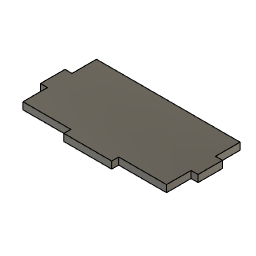
Assemble_Habits v10 (Autodesk Fusion 360 archive; units mm, degrees)
design "tray_front2_43x25_trans_2mm"
Autodesk Fusion 360 part; units mm, degrees
note: some values were not read from the file. Set by a fixed rule: which face or edge a step refers to.
(part 1 of 2)
sketch "Sketch1" plane through (0, 0, 0) normal (0, 0, 1) x (1, 0, 0)
  line L0 (0, 0) -> (41, 0)
  line L1 (41, 0) -> (41, -21)
  line L2 (41, -21) -> (0, -21)
  line L3 (0, -21) -> (0, 0)
  line L4 (0, -21) -> (0, -14)
  line L5 (0, -14) -> (-2, -14)
  line L6 (-2, -14) -> (-2, -7)
  line L7 (-2, -7) -> (0, -7)
  line L8 (0, -7) -> (0, -14)
  line L9 (41, -21) -> (41, -14)
  line L10 (41, -14) -> (43, -14)
  line L11 (43, -14) -> (43, -7)
  line L12 (43, -7) -> (41, -7)
  line L13 (41, -7) -> (41, -14)
  line L14 (0, -21) -> (13.67, -21)
  line L15 (13.67, -21) -> (27.34, -21)
  line L16 (27.34, -21) -> (27.34, -23)
  line L17 (27.34, -23) -> (13.67, -23)
  line L18 (13.67, -23) -> (13.67, -21)
  dimension "d1" = 41
  dimension "d2" = 21
  dimension "d5" = 7
  dimension "d6" = 2
  dimension "d7" = 7
  dimension "d8" = 7
  dimension "d9" = 2
  dimension "d10" = 7
  dimension "d11" = 13.67
  dimension "d12" = 13.67
  dimension "d13" = 2
  constraint horizontal L0
  constraint vertical L1
  constraint horizontal L2
  constraint vertical L3
  constraint coincident L0.start L3.end
  constraint perpendicular L2 L4
  constraint horizontal L5
  constraint vertical L6
  constraint horizontal L7
  constraint vertical L8
  constraint perpendicular L2 L9
  constraint horizontal L10
  constraint vertical L11
  constraint horizontal L12
  constraint vertical L13
  constraint perpendicular L3 L14
  constraint horizontal L15
  constraint vertical L16
  constraint horizontal L17
  constraint vertical L18
  measures "d1" distance of L0.start L0.end
  measures "d2" distance of L0.start L2.end
  measures "d5" distance of L2.end L4.end
  measures "d6" distance of L4.end L5.end
  measures "d7" distance of L4.end L7.end
  measures "d8" distance of L1.end L9.end
  measures "d9" distance of L9.end L10.end
  measures "d10" distance of L9.end L12.end
  measures "d11" distance of L2.end L14.end
  measures "d12" distance of L14.end L15.end
  measures "d13" distance of L14.end L17.end
extrude "Extrude1" add sketch "Sketch1" along normal blind 2

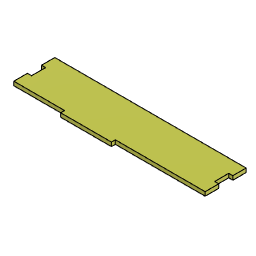
design "tray_side2_98x23_trans_2mm"
Autodesk Fusion 360 part; units mm, degrees
sketch "Sketch1" plane through (0, 0, 0) normal (0, 0, 1) x (1, 0, 0)
  line L0 (0, 0) -> (98, 0)
  line L1 (98, 0) -> (98, -21)
  line L2 (98, -21) -> (0, -21)
  line L3 (0, -21) -> (0, 0)
  line L4 (0, -21) -> (0, -14)
  line L5 (0, -14) -> (2.1, -14)
  line L6 (2.1, -14) -> (2.1, -6.8)
  line L7 (2.1, -6.8) -> (0, -6.8)
  line L8 (0, -6.8) -> (0, -14)
  line L9 (98, -21) -> (98, -14)
  line L10 (98, -14) -> (95.9, -14)
  line L11 (95.9, -14) -> (95.9, -6.8)
  line L12 (95.9, -6.8) -> (98, -6.8)
  line L13 (98, -6.8) -> (98, -14)
  line L14 (0, -21) -> (26, -21)
  line L15 (26, -21) -> (52, -21)
  line L16 (52, -21) -> (52, -23)
  line L17 (52, -23) -> (26, -23)
  line L18 (26, -23) -> (26, -21)
  dimension "d1" = 98
  dimension "d2" = 21
  dimension "d5" = 7
  dimension "d6" = 2.1
  dimension "d7" = 7.2
  dimension "d8" = 7
  dimension "d9" = 2.1
  dimension "d10" = 7.2
  dimension "d11" = 26
  dimension "d12" = 26
  dimension "d13" = 2
  constraint horizontal L0
  constraint vertical L1
  constraint horizontal L2
  constraint vertical L3
  constraint coincident L0.start L3.end
  constraint perpendicular L2 L4
  constraint horizontal L5
  constraint vertical L6
  constraint horizontal L7
  constraint vertical L8
  constraint perpendicular L2 L9
  constraint horizontal L10
  constraint vertical L11
  constraint horizontal L12
  constraint vertical L13
  constraint perpendicular L3 L14
  constraint horizontal L15
  constraint vertical L16
  constraint horizontal L17
  constraint vertical L18
  measures "d1" distance of L0.start L0.end
  measures "d2" distance of L0.start L2.end
  measures "d5" distance of L2.end L4.end
  measures "d6" distance of L4.end L5.end
  measures "d7" distance of L4.end L7.end
  measures "d8" distance of L1.end L9.end
  measures "d9" distance of L9.end L10.end
  measures "d10" distance of L9.end L12.end
  measures "d11" distance of L2.end L14.end
  measures "d12" distance of L14.end L15.end
  measures "d13" distance of L14.end L17.end
extrude "Extrude1" add sketch "Sketch1" along normal blind 2 contours L0 L1 L2 L3 L4 L5 L6 L7 L9 L10 L11 L12 L14 L15 | L2 L15 L16 L17 L18

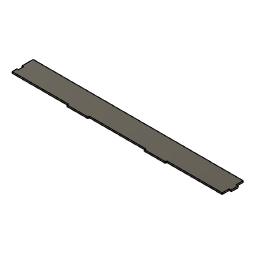
design "tray_side_302x32_trans_2mm"
Autodesk Fusion 360 part; units mm, degrees
sketch "Sketch1" plane through (0, 0, 0) normal (0, 0, 1) x (1, 0, 0)
  line L0 (0, 0) -> (299, 0)
  line L1 (299, 0) -> (299, -30)
  line L2 (299, -30) -> (0, -30)
  line L3 (0, -30) -> (0, 0)
  line L4 (0, -30) -> (0, -23)
  line L5 (0, -23) -> (2.1, -23)
  line L6 (2.1, -23) -> (2.1, -15.8)
  line L7 (2.1, -15.8) -> (0, -15.8)
  line L8 (0, -15.8) -> (0, -23)
  line L9 (299, -30) -> (299, -20)
  line L10 (299, -20) -> (302, -20)
  line L11 (302, -20) -> (302, -10)
  line L12 (302, -10) -> (299, -10)
  line L13 (299, -10) -> (299, -20)
  line L14 (0, -30) -> (80, -30)
  line L15 (80, -30) -> (110, -30)
  line L16 (110, -30) -> (110, -32)
  line L17 (110, -32) -> (80, -32)
  line L18 (80, -32) -> (80, -30)
  line L19 (110, -30) -> (190.2, -30)
  line L20 (190.2, -30) -> (220.2, -30)
  line L21 (220.2, -30) -> (220.2, -32)
  line L22 (220.2, -32) -> (190.2, -32)
  line L23 (190.2, -32) -> (190.2, -30)
  dimension "d1" = 299
  dimension "d2" = 30
  dimension "d5" = 7
  dimension "d6" = 2.1
  dimension "d7" = 7.2
  dimension "d8" = 10
  dimension "d9" = 3
  dimension "d10" = 10
  dimension "d11" = 80
  dimension "d12" = 30
  dimension "d13" = 2
  dimension "d14" = 80.2
  dimension "d15" = 30
  dimension "d16" = 2
  constraint horizontal L0
  constraint vertical L1
  constraint horizontal L2
  constraint vertical L3
  constraint coincident L0.start L3.end
  constraint perpendicular L2 L4
  constraint horizontal L5
  constraint vertical L6
  constraint horizontal L7
  constraint vertical L8
  constraint perpendicular L2 L9
  constraint horizontal L10
  constraint vertical L11
  constraint horizontal L12
  constraint vertical L13
  constraint perpendicular L4 L14
  constraint horizontal L15
  constraint vertical L16
  constraint horizontal L17
  constraint vertical L18
  constraint perpendicular L16 L19
  constraint horizontal L20
  constraint vertical L21
  constraint horizontal L22
  constraint vertical L23
  measures "d1" distance of L0.start L0.end
  measures "d2" distance of L0.start L2.end
  measures "d5" distance of L2.end L4.end
  measures "d6" distance of L4.end L5.end
  measures "d7" distance of L4.end L7.end
  measures "d8" distance of L1.end L9.end
  measures "d9" distance of L9.end L10.end
  measures "d10" distance of L9.end L12.end
  measures "d11" distance of L2.end L14.end
  measures "d12" distance of L14.end L15.end
  measures "d13" distance of L14.end L17.end
  measures "d14" distance of L15.end L19.end
  measures "d15" distance of L19.end L20.end
  measures "d16" distance of L19.end L22.end
extrude "Extrude1" add sketch "Sketch1" along normal blind 2 contours L0 L1 L2 L3 L4 L5 L6 L7 L9 L13 L14 L15 L19 L20 | L1 L10 L11 L12 L13 | L2 L15 L16 L17 L18 | L2 L20 L21 L22 L23

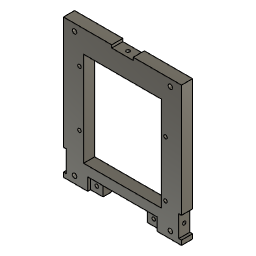
design "Front_holder"
Autodesk Fusion 360 part; units mm, degrees
sketch "Sketch1" plane through (0, 0, 0) normal (0, 1, 0) x (1, 0, 0)
  line L0 (0, 0) -> (85, 0)
  line L1 (85, 0) -> (85, -100)
  line L2 (85, -100) -> (0, -100)
  line L3 (0, -100) -> (0, 0)
  line L4 (85, 0) -> (85, -3.25)
  line L5 (85, -3.25) -> (83, -3.25)
  line L6 (83, -3.25) -> (83, -18.75)
  line L7 (83, -18.75) -> (85, -18.75)
  line L8 (85, -18.75) -> (85, -3.25)
  line L9 (0, 0) -> (0, -3.25)
  line L10 (0, -3.25) -> (2, -3.25)
  line L11 (2, -3.25) -> (2, -18.75)
  line L12 (2, -18.75) -> (0, -18.75)
  line L13 (0, -18.75) -> (0, -3.25)
  line L14 (0, -100) -> (34.75, -100)
  line L15 (34.75, -100) -> (50.25, -100)
  line L16 (50.25, -100) -> (50.25, -98)
  line L17 (50.25, -98) -> (34.75, -98)
  line L18 (34.75, -98) -> (34.75, -100)
  line L19 (0, -100) -> (8.5, -100)
  line L20 (8.5, -100) -> (8.5, -90)
  line L21 (8.5, -90) -> (0, -90)
  line L22 (0, -90) -> (0, -100)
  line L23 (8.5, -90) -> (76.5, -90)
  line L24 (76.5, -90) -> (76.5, -10)
  line L25 (76.5, -10) -> (8.5, -10)
  line L26 (8.5, -10) -> (8.5, -90)
  circle A0 centre (8, -95) radius 1.6
  circle A1 centre (77, -95) radius 1.6
  circle A2 centre (8, -5) radius 1.6
  circle A3 centre (77, -5) radius 1.6
  circle A4 centre (11.5, -35) radius 1.25
  circle A5 centre (11.5, -75) radius 1.25
  circle A6 centre (73.5, -22) radius 1.25
  line L27 (8.5, -90) -> (14.5, -90)
  line L28 (14.5, -90) -> (14.5, -84)
  line L29 (14.5, -84) -> (8.5, -84)
  line L30 (8.5, -84) -> (8.5, -90)
  line L31 (14.5, -84) -> (70.5, -84)
  line L32 (70.5, -84) -> (70.5, -16)
  line L33 (70.5, -16) -> (14.5, -16)
  line L34 (14.5, -16) -> (14.5, -84)
  circle A7 centre (73.5, -62) radius 1.25
  line L35 (42.5, 0) -> (67.5, 0)
  line L36 (67.5, 0) -> (17.5, 0)
  line L37 (17.5, 0) -> (17.5, -9)
  line L38 (17.5, -9) -> (67.5, -9)
  line L39 (67.5, -9) -> (67.5, 0)
  line L40 (17.5, 0) -> (26.5, 0)
  line L41 (67.5, 0) -> (58.5, 0)
  line L42 (26.5, 0) -> (26.5, -9)
  line L43 (58.5, 0) -> (58.5, -9)
  circle A8 centre (22, -4.5) radius 1.25
  circle A9 centre (63, -4.5) radius 1.25
  dimension "d1" = 85
  dimension "d2" = 100
  dimension "d25" = 3.25
  dimension "d26" = 2
  dimension "d27" = 15.5
  dimension "d28" = 3.25
  dimension "d29" = 2
  dimension "d30" = 15.5
  dimension "d31" = 34.75
  dimension "d32" = 15.5
  dimension "d33" = 2
  dimension "d45" = 8.5
  dimension "d46" = 10
  dimension "d47" = 68
  dimension "d48" = 80
  dimension "d49" = 3.2
  dimension "d50" = 8
  dimension "d51" = 3.2
  dimension "d52" = 8
  dimension "d53" = 3.2
  dimension "d54" = 5
  dimension "d55" = 3.2
  dimension "d56" = 8
  dimension "d57" = 2.5
  dimension "d58" = 25
  dimension "d59" = 3
  dimension "d60" = 2.5
  dimension "d61" = 65
  dimension "d62" = 2.5
  dimension "d63" = 65
  dimension "d64" = 12
  dimension "d161" = 6
  dimension "d162" = 6
  dimension "d163" = 56
  dimension "d164" = 68
  dimension "d167" = 8
  dimension "d168" = 5
  dimension "d213" = 2.5
  dimension "d214" = 40
  dimension "d215" = 25
  dimension "d216" = 50
  dimension "d217" = 9
  dimension "d218" = 9
  dimension "d219" = 9
  dimension "d223" = 2.5
  dimension "d224" = 2.5
  dimension "d225" = 4.5
  dimension "d226" = 4.5
  constraint horizontal L0
  constraint vertical L1
  constraint horizontal L2
  constraint vertical L3
  constraint coincident L0.start L3.end
  constraint perpendicular L0 L4
  constraint horizontal L5
  constraint vertical L6
  constraint horizontal L7
  constraint vertical L8
  constraint perpendicular L0 L9
  constraint horizontal L10
  constraint vertical L11
  constraint horizontal L12
  constraint vertical L13
  constraint perpendicular L3 L14
  constraint horizontal L15
  constraint vertical L16
  constraint horizontal L17
  constraint vertical L18
  constraint horizontal L19
  constraint vertical L20
  constraint horizontal L21
  constraint vertical L22
  constraint horizontal L23
  constraint vertical L24
  constraint horizontal L25
  constraint vertical L26
  constraint horizontal L27
  constraint vertical L28
  constraint horizontal L29
  constraint vertical L30
  constraint horizontal L31
  constraint vertical L32
  constraint horizontal L33
  constraint vertical L34
  constraint midpoint L0 L35.start
  constraint parallel L0 L35
  constraint horizontal L36
  constraint vertical L37
  constraint horizontal L38
  constraint vertical L39
  constraint perpendicular L37 L40
  constraint perpendicular L39 L41
  constraint coincident L38 L42.end
  constraint perpendicular L38 L42
  constraint coincident L38 L43.end
  constraint perpendicular L38 L43
  measures "d1" distance of L0.start L0.end
  measures "d2" distance of L0.start L2.end
  measures "d25" distance of L0.end L4.end
  measures "d26" distance of L4.end L5.end
  measures "d27" distance of L4.end L7.end
  measures "d28" distance of L0.start L9.end
  measures "d29" distance of L9.end L10.end
  measures "d30" distance of L9.end L12.end
  measures "d31" distance of L2.end L14.end
  measures "d32" distance of L14.end L15.end
  measures "d33" distance of L14.end L17.end
  measures "d45" distance of L2.end L19.end
  measures "d46" distance of L2.end L21.end
  measures "d47" distance of L20.end L23.end
  measures "d48" distance of L20.end L25.end
  measures "d49" diameter of A0
  measures "d50" distance of L3 A0.centre
  measures "d51" diameter of A1
  measures "d52" distance of L1 A1.centre
  measures "d53" diameter of A2
  measures "d54" distance of L0 A2.centre
  measures "d55" diameter of A3
  measures "d56" distance of L8 A3.centre
  measures "d57" diameter of A4
  measures "d58" distance of L25 A4.centre
  measures "d59" distance of L26 A4.centre
  measures "d60" diameter of A5
  measures "d61" distance of L25 A5.centre
  measures "d62" diameter of A6
  measures "d63" distance of L26 A6.centre
  measures "d64" distance of L25 A6.centre
  measures "d161" distance of L20.end L27.end
  measures "d162" distance of L20.end L29.end
  measures "d163" distance of L28.end L31.end
  measures "d164" distance of L28.end L33.end
  measures "d167" distance of L13 A2.centre
  measures "d168" distance of L0 A3.centre
  measures "d213" diameter of A7
  measures "d214" distance of A6.centre A7.centre
  measures "d215" distance of L35.start L35.end
  measures "d216" distance of L35.end L36.end
  measures "d217" distance of L35.end L38.end
  measures "d218" distance of L36.end L40.end
  measures "d219" distance of L35.end L41.end
  measures "d223" diameter of A8
  measures "d224" diameter of A9
  measures "d225" distance of L37 A8.centre
  measures "d226" distance of L39 A9.centre
extrude "Extrude1" add sketch "Sketch1" along normal blind 8 contours L23 L26 L27 L28 L29 L30 | L0 L1 L2 L3 L4 L5 L6 L7 L9 L10 L11 L12 L14 L16 L17 L18 L20 L21 A0 L37 L38 L39 | L2 L3 L14 L19 L20 L21 L22 A0 | L23 L24 L25 L26 L28 L29
hole "Hole1" at (42.5, 4, 98) direction (0, 0, -1) diameter 2.5 depth 12 tip angle 180
hole "Hole2" at (83, 4, 11) direction (-1, 0, 0) diameter 2.5 depth 12 tip angle 180
hole "Hole3" at (2, 4, 11) direction (1, 0, 0) diameter 2.5 depth 12 tip angle 180
extrude "Extrude7" add sketch "Sketch1" along normal blind 6 from surface at 2 contours L0 L36 L37 L38 L40 L42 | L0 L35 L36 L38 L39 L41 L43

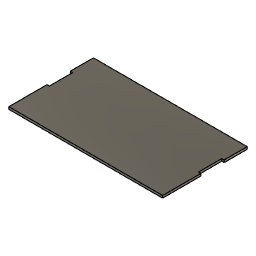
design "cage_back_200x110_trans_3mm"
Autodesk Fusion 360 part; units mm, degrees
sketch "Sketch1" plane through (0, 0, 0) normal (0, 0, 1) x (1, 0, 0)
  line L0 (0, 0) -> (200, 0)
  line L1 (200, 0) -> (200, -110)
  line L2 (200, -110) -> (0, -110)
  line L3 (0, -110) -> (0, 0)
  line L4 (0, 0) -> (0, -30)
  line L5 (0, -30) -> (3.1, -30)
  line L6 (3.1, -30) -> (3.1, -60.2)
  line L7 (3.1, -60.2) -> (0, -60.2)
  line L8 (0, -60.2) -> (0, -30)
  line L9 (200, 0) -> (200, -30)
  line L10 (200, -30) -> (196.9, -30)
  line L11 (196.9, -30) -> (196.9, -60.2)
  line L12 (196.9, -60.2) -> (200, -60.2)
  line L13 (200, -60.2) -> (200, -30)
  dimension "d1" = 200
  dimension "d2" = 110
  dimension "d5" = 30
  dimension "d6" = 3.1
  dimension "d7" = 30.2
  dimension "d8" = 30
  dimension "d9" = 3.1
  dimension "d10" = 30.2
  constraint horizontal L0
  constraint vertical L1
  constraint horizontal L2
  constraint vertical L3
  constraint coincident L0.start L3.end
  constraint parallel L3 L4
  constraint horizontal L5
  constraint vertical L6
  constraint horizontal L7
  constraint vertical L8
  constraint perpendicular L0 L9
  constraint horizontal L10
  constraint vertical L11
  constraint horizontal L12
  constraint vertical L13
  measures "d1" distance of L0.start L0.end
  measures "d2" distance of L0.start L2.end
  measures "d5" distance of L0.start L4.end
  measures "d6" distance of L4.end L5.end
  measures "d7" distance of L4.end L7.end
  measures "d8" distance of L0.end L9.end
  measures "d9" distance of L9.end L10.end
  measures "d10" distance of L9.end L12.end
extrude "Extrude1" add sketch "Sketch1" along normal blind 3 contours L0 L1 L2 L3 L4 L5 L6 L7 L9 L10 L11 L12

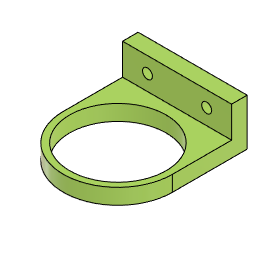
design "Tube_holder"
Autodesk Fusion 360 part; units mm, degrees
sketch "Sketch1" plane through (0, 0, 0) normal (0, 0, 1) x (1, 0, 0)
  circle A0 centre (0, 0) radius 15.5
  circle A1 centre (0, 0) radius 17.5
  line L0 (0, 0) -> (17.5, 0)
  line L1 (0, 0) -> (-17.5, 0)
  line L2 (-17.5, 0) -> (-17.5, 24)
  line L3 (17.5, 0) -> (17.5, 24)
  line L4 (-17.5, 24) -> (17.5, 24)
  line L5 (-17.5, 24) -> (-17.5, 19)
  line L6 (-17.5, 19) -> (17.5, 19)
  dimension "d1" = 31
  dimension "d2" = 35
  dimension "d3" = 24
  dimension "d4" = 24
  dimension "d9" = 5
  constraint coincident A0.centre A1.centre
  constraint concentric A0 A1
  constraint coincident A1 L0.end
  constraint horizontal L0
  constraint coincident A1 L1.end
  constraint parallel L0 L1
  constraint perpendicular L1 L2
  constraint perpendicular L0 L3
  constraint perpendicular L4 L5
  constraint coincident L3 L6.end
  constraint perpendicular L3 L6
  measures "d1" diameter of A0
  measures "d2" diameter of A1
  measures "d3" distance of L1.end L2.end
  measures "d4" distance of L0.end L3.end
  measures "d9" distance of L2.end L5.end
extrude "Extrude1" add sketch "Sketch1" along normal blind 5 contours A0 A1 L0 L1 | A0 A1 L0 L1 | A1 L2 L3 L6 | L2 L3 L4 L5 L6
extrude "Extrude2" add sketch "Sketch1" along normal blind 15 contours L2 L3 L4 L5 L6
sketch "Sketch2" plane through (0, 19, 0) normal (0, -1, 0) x (1, 0, 0)
  line L0 (-17.5, 5) -> (17.5, 5)
  line L1 (17.5, 5) -> (17.5, 15)
  line L2 (17.5, 15) -> (-17.5, 15)
  line L3 (-17.5, 15) -> (-17.5, 5)
  circle A0 centre (-9.5, 10) radius 1.6
  circle A1 centre (9.5, 10) radius 1.6
  dimension "d10" = 3.2
  dimension "d11" = 3.2
  dimension "d12" = 8
  dimension "d13" = 8
  measures "d10" diameter of A0
  measures "d11" diameter of A1
  measures "d12" distance of L3 A0.centre
  measures "d13" distance of L1 A1.centre
extrude "Extrude3" cut sketch "Sketch2" against normal blind 5 contours A0 | A1

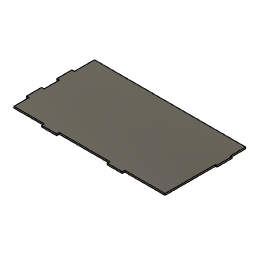
design "cage_side_308x165_blk_3mm"
Autodesk Fusion 360 part; units mm, degrees
sketch "Sketch1" plane through (0, 0, 0) normal (0, 0, 1) x (1, 0, 0)
  line L0 (0, 0) -> (300, 0)
  line L1 (300, 0) -> (300, -160)
  line L2 (300, -160) -> (0, -160)
  line L3 (0, -160) -> (0, 0)
  line L4 (0, -160) -> (60, -160)
  line L5 (60, -160) -> (90, -160)
  line L6 (90, -160) -> (90, -165)
  line L7 (90, -165) -> (60, -165)
  line L8 (60, -165) -> (60, -160)
  line L9 (90, -160) -> (190.2, -160)
  line L10 (190.2, -160) -> (220.2, -160)
  line L11 (220.2, -160) -> (220.2, -165)
  line L12 (220.2, -165) -> (190.2, -165)
  line L13 (190.2, -165) -> (190.2, -160)
  line L14 (0, -160) -> (0, -130)
  line L15 (0, -130) -> (-5, -130)
  line L16 (-5, -130) -> (-5, -100)
  line L17 (-5, -100) -> (0, -100)
  line L18 (0, -100) -> (0, -130)
  line L19 (0, -100) -> (0, -69.8)
  line L20 (0, -69.8) -> (-5, -69.8)
  line L21 (-5, -69.8) -> (-5, -39.8)
  line L22 (-5, -39.8) -> (0, -39.8)
  line L23 (0, -39.8) -> (0, -69.8)
  line L24 (300, 0) -> (300, -30)
  line L25 (300, -30) -> (303, -30)
  line L26 (303, -30) -> (303, -60)
  line L27 (303, -60) -> (300, -60)
  line L28 (300, -60) -> (300, -30)
  dimension "d1" = 300
  dimension "d2" = 160
  dimension "d5" = 60
  dimension "d6" = 30
  dimension "d7" = 5
  dimension "d8" = 100.2
  dimension "d9" = 30
  dimension "d10" = 5
  dimension "d11" = 30
  dimension "d12" = 5
  dimension "d13" = 30
  dimension "d14" = 30.2
  dimension "d15" = 5
  dimension "d16" = 30
  dimension "d17" = 30
  dimension "d18" = 3
  dimension "d19" = 30
  constraint horizontal L0
  constraint vertical L1
  constraint horizontal L2
  constraint vertical L3
  constraint coincident L0.start L3.end
  constraint perpendicular L3 L4
  constraint horizontal L5
  constraint vertical L6
  constraint horizontal L7
  constraint vertical L8
  constraint perpendicular L6 L9
  constraint horizontal L10
  constraint vertical L11
  constraint horizontal L12
  constraint vertical L13
  constraint perpendicular L4 L14
  constraint horizontal L15
  constraint vertical L16
  constraint horizontal L17
  constraint vertical L18
  constraint perpendicular L17 L19
  constraint horizontal L20
  constraint vertical L21
  constraint horizontal L22
  constraint vertical L23
  constraint perpendicular L0 L24
  constraint horizontal L25
  constraint vertical L26
  constraint horizontal L27
  constraint vertical L28
  measures "d1" distance of L0.start L0.end
  measures "d2" distance of L0.start L2.end
  measures "d5" distance of L2.end L4.end
  measures "d6" distance of L4.end L5.end
  measures "d7" distance of L4.end L7.end
  measures "d8" distance of L5.end L9.end
  measures "d9" distance of L9.end L10.end
  measures "d10" distance of L9.end L12.end
  measures "d11" distance of L2.end L14.end
  measures "d12" distance of L14.end L15.end
  measures "d13" distance of L14.end L17.end
  measures "d14" distance of L17.end L19.end
  measures "d15" distance of L19.end L20.end
  measures "d16" distance of L19.end L22.end
  measures "d17" distance of L0.end L24.end
  measures "d18" distance of L24.end L25.end
  measures "d19" distance of L24.end L27.end
extrude "Extrude1" add sketch "Sketch1" along normal blind 3

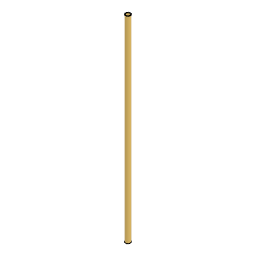
design "Lickport"
Autodesk Fusion 360 part; units mm, degrees
sketch "Sketch1" plane through (0, 0, 0) normal (0, 0, 1) x (1, 0, 0)
  circle A0 centre (0, 0) radius 0.75
  circle A1 centre (0, 0) radius 0.6
  dimension "d1" = 1.5
  dimension "d4" = 1.2
  constraint coincident A0.centre A1.centre
  constraint concentric A0 A1
  measures "d1" diameter of A0
  measures "d4" diameter of A1
extrude "Extrude2" add sketch "Sketch1" along normal blind 60

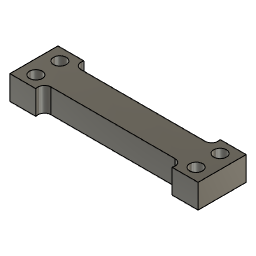
design "weight_Load cell"
Autodesk Fusion 360 part; units mm, degrees
sketch "Sketch1" plane through (0, 0, 0) normal (0, 0, 1) x (1, 0, 0)
  line L0 (0, 0) -> (47, 0)
  line L1 (47, 0) -> (47, -12)
  line L2 (47, -12) -> (0, -12)
  line L3 (0, -12) -> (0, 0)
  circle A0 centre (3.5, -3) radius 1.6
  circle A1 centre (3.5, -9) radius 1.6
  circle A2 centre (43.5, -3) radius 1.6
  circle A3 centre (43.5, -9) radius 1.6
  line L4 (23.5, 0) -> (6.5, 0)
  line L5 (23.5, -2.25) -> (8, -2.25)
  arc A4 (6.5, 0) -> (8, -2.25) centre (8, -0.625) ccw
  line L6 (23.5, -2.25) -> (39, -2.25)
  line L7 (23.5, 0) -> (40.5, 0)
  arc A5 (39, -2.25) -> (40.5, 0) centre (39, -0.625) ccw
  line L8 (23.5, -9.75) -> (8, -9.75)
  line L9 (23.5, -9.75) -> (39, -9.75)
  line L10 (23.5, -12) -> (40.5, -12)
  line L11 (23.5, -12) -> (6.5, -12)
  arc A6 (8, -9.75) -> (6.5, -12) centre (8, -11.375) ccw
  arc A7 (40.5, -12) -> (39, -9.75) centre (39, -11.375) ccw
  dimension "d2" = 47
  dimension "d3" = 12
  dimension "d4" = 40
  dimension "d5" = 6
  dimension "d6" = 3.2
  dimension "d7" = 3.2
  dimension "d8" = 3.2
  dimension "d9" = 3.2
  dimension "d12" = 17
  dimension "d13" = 15.5
  dimension "d14" = 15.5
  dimension "d15" = 17
  dimension "d17" = 15.5
  dimension "d18" = 15.5
  dimension "d19" = 17
  dimension "d20" = 17
  constraint horizontal L0
  constraint vertical L1
  constraint horizontal L2
  constraint vertical L3
  constraint coincident L0.start L3.end
  constraint midpoint L0 L4.start
  constraint parallel L0 L4
  constraint tangent L5 A4
  constraint parallel L0 L7
  constraint tangent L6 A5
  constraint midpoint L2 L10.start
  constraint parallel L2 L10
  constraint parallel L2 L11
  constraint tangent L8 A6
  constraint tangent L9 A7
  measures "d2" distance of L0.start L0.end
  measures "d3" distance of L0.start L2.end
  measures "d4" distance of A0.centre A2.centre
  measures "d5" distance of A0.centre A1.centre
  measures "d6" diameter of A0
  measures "d7" diameter of A1
  measures "d8" diameter of A2
  measures "d9" diameter of A3
  measures "d12" distance of L4.start L4.end
  measures "d13" distance of L5.start L5.end
  measures "d14" distance of L5.start L6.end
  measures "d15" distance of L4.start L7.end
  measures "d17" distance of L8.start L8.end
  measures "d18" distance of L8.start L9.end
  measures "d19" distance of L10.start L10.end
  measures "d20" distance of L10.start L11.end
extrude "Extrude1" add sketch "Sketch1" along normal blind 6 contours L0 L1 L2 L3 L5 A4 L6 A5 L8 L9 A6 A7
equation "d13 = 17 mm - 1.5 mm"

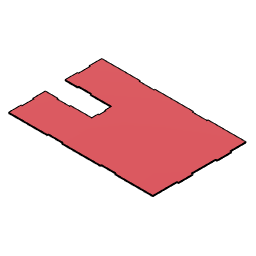
design "tray_bottom_302x193_trans_2mm"
Autodesk Fusion 360 part; units mm, degrees
sketch "Sketch1" plane through (0, 0, 0) normal (0, 0, 1) x (1, 0, 0)
  line L0 (0, 0) -> (299, 0)
  line L1 (299, 0) -> (299, -193)
  line L2 (299, -193) -> (0, -193)
  line L3 (0, -193) -> (0, 0)
  line L4 (0, -193) -> (80, -193)
  line L5 (80, -193) -> (110.2, -193)
  line L6 (110.2, -193) -> (110.2, -190.9)
  line L7 (110.2, -190.9) -> (80, -190.9)
  line L8 (80, -190.9) -> (80, -193)
  line L9 (110.2, -193) -> (190.2, -193)
  line L10 (190.2, -193) -> (220.4, -193)
  line L11 (220.4, -193) -> (220.4, -190.9)
  line L12 (220.4, -190.9) -> (190.2, -190.9)
  line L13 (190.2, -190.9) -> (190.2, -193)
  line L14 (0, 0) -> (80, 0)
  line L15 (80, 0) -> (110.2, 0)
  line L16 (110.2, 0) -> (110.2, -2.1)
  line L17 (110.2, -2.1) -> (80, -2.1)
  line L18 (80, -2.1) -> (80, 0)
  line L19 (110.2, 0) -> (190.2, 0)
  line L20 (190.2, 0) -> (220.4, 0)
  line L21 (220.4, 0) -> (220.4, -2.1)
  line L22 (220.4, -2.1) -> (190.2, -2.1)
  line L23 (190.2, -2.1) -> (190.2, 0)
  line L24 (299, -193) -> (299, -143)
  line L25 (299, -143) -> (302, -143)
  line L26 (302, -143) -> (302, -113)
  line L27 (302, -113) -> (299, -113)
  line L28 (299, -113) -> (299, -143)
  line L29 (299, -113) -> (299, -62.8)
  line L30 (299, -62.8) -> (302, -62.8)
  line L31 (302, -62.8) -> (302, -32.8)
  line L32 (302, -32.8) -> (299, -32.8)
  line L33 (299, -32.8) -> (299, -62.8)
  line L34 (96, -116.8364) -> (0, -116.8364)
  line L35 (0, -116.8364) -> (0, -75.8364)
  line L36 (0, -75.8364) -> (96, -75.8364)
  line L37 (96, -75.8364) -> (96, -116.8364)
  line L38 (96, -116.8364) -> (0, -75.8364) construction
  line L39 (0, -116.8364) -> (96, -75.8364) construction
  line L40 (0, -193) -> (0, -167)
  line L41 (0, -167) -> (2.1, -167)
  line L42 (2.1, -167) -> (2.1, -142.8)
  line L43 (2.1, -142.8) -> (0, -142.8)
  line L44 (0, -142.8) -> (0, -167)
  line L45 (0, 0) -> (0, -26)
  line L46 (0, -26) -> (2.1, -26)
  line L47 (2.1, -26) -> (2.1, -50)
  line L48 (2.1, -50) -> (0, -50)
  line L49 (0, -50) -> (0, -26)
  line L50 (0, -116.8364) -> (26, -116.8364)
  line L51 (26, -116.8364) -> (52.2, -116.8364)
  line L52 (52.2, -116.8364) -> (52.2, -118.9364)
  line L53 (52.2, -118.9364) -> (26, -118.9364)
  line L54 (26, -118.9364) -> (26, -116.8364)
  line L55 (0, -75.8364) -> (26, -75.8364)
  line L56 (26, -75.8364) -> (52.2, -75.8364)
  line L57 (52.2, -75.8364) -> (52.2, -73.7364)
  line L58 (52.2, -73.7364) -> (26, -73.7364)
  line L59 (26, -73.7364) -> (26, -75.8364)
  line L60 (96, -75.8364) -> (96, -89.5064)
  line L61 (96, -89.5064) -> (98.1, -89.5064)
  line L62 (98.1, -89.5064) -> (98.1, -103.3764)
  line L63 (98.1, -103.3764) -> (96, -103.3764)
  line L64 (96, -103.3764) -> (96, -89.5064)
  point P0 (48, -96.3364)
  dimension "d1" = 299
  dimension "d2" = 193
  dimension "d17" = 80
  dimension "d18" = 30.2
  dimension "d19" = 2.1
  dimension "d20" = 80
  dimension "d21" = 30.2
  dimension "d22" = 2.1
  dimension "d23" = 80
  dimension "d24" = 30.2
  dimension "d25" = 2.1
  dimension "d26" = 80
  dimension "d27" = 30.2
  dimension "d28" = 2.1
  dimension "d29" = 50
  dimension "d30" = 3
  dimension "d31" = 30
  dimension "d32" = 50.2
  dimension "d33" = 3
  dimension "d34" = 30
  dimension "d36" = 41
  dimension "d37" = 48
  dimension "d38" = 26
  dimension "d39" = 2.1
  dimension "d40" = 24.2
  dimension "d41" = 26
  dimension "d42" = 2.1
  dimension "d43" = 24
  dimension "d44" = 26
  dimension "d45" = 26.2
  dimension "d46" = 2.1
  dimension "d47" = 26
  dimension "d48" = 26.2
  dimension "d49" = 2.1
  dimension "d50" = 13.67
  dimension "d51" = 2.1
  dimension "d52" = 13.87
  dimension "d53" = 96
  constraint horizontal L0
  constraint vertical L1
  constraint horizontal L2
  constraint vertical L3
  constraint coincident L0.start L3.end
  constraint perpendicular L3 L4
  constraint horizontal L5
  constraint vertical L6
  constraint horizontal L7
  constraint vertical L8
  constraint perpendicular L6 L9
  constraint horizontal L10
  constraint vertical L11
  constraint horizontal L12
  constraint vertical L13
  constraint perpendicular L3 L14
  constraint horizontal L15
  constraint vertical L16
  constraint horizontal L17
  constraint vertical L18
  constraint perpendicular L16 L19
  constraint horizontal L20
  constraint vertical L21
  constraint horizontal L22
  constraint vertical L23
  constraint perpendicular L2 L24
  constraint horizontal L25
  constraint vertical L26
  constraint horizontal L27
  constraint vertical L28
  constraint perpendicular L27 L29
  constraint horizontal L30
  constraint vertical L31
  constraint horizontal L32
  constraint vertical L33
  constraint horizontal L34
  constraint perpendicular L34 L35
  constraint parallel L34 L36
  constraint parallel L35 L37
  constraint coincident L38 P0
  constraint coincident L39 P0
  constraint perpendicular L4 L40
  constraint horizontal L41
  constraint vertical L42
  constraint horizontal L43
  constraint vertical L44
  constraint perpendicular L14 L45
  constraint horizontal L46
  constraint vertical L47
  constraint horizontal L48
  constraint vertical L49
  constraint perpendicular L3 L50
  constraint horizontal L51
  constraint vertical L52
  constraint horizontal L53
  constraint vertical L54
  constraint perpendicular L35 L55
  constraint horizontal L56
  constraint vertical L57
  constraint horizontal L58
  constraint vertical L59
  constraint perpendicular L36 L60
  constraint horizontal L61
  constraint vertical L62
  constraint horizontal L63
  constraint vertical L64
  measures "d1" distance of L0.start L0.end
  measures "d2" distance of L0.start L2.end
  measures "d17" distance of L2.end L4.end
  measures "d18" distance of L4.end L5.end
  measures "d19" distance of L4.end L7.end
  measures "d20" distance of L5.end L9.end
  measures "d21" distance of L9.end L10.end
  measures "d22" distance of L9.end L12.end
  measures "d23" distance of L0.start L14.end
  measures "d24" distance of L14.end L15.end
  measures "d25" distance of L14.end L17.end
  measures "d26" distance of L15.end L19.end
  measures "d27" distance of L19.end L20.end
  measures "d28" distance of L19.end L22.end
  measures "d29" distance of L1.end L24.end
  measures "d30" distance of L24.end L25.end
  measures "d31" distance of L24.end L27.end
  measures "d32" distance of L27.end L29.end
  measures "d33" distance of L29.end L30.end
  measures "d34" distance of L29.end L32.end
  measures "d36" distance of L34.end L35.end
  measures "d37" distance of L3 P0
  measures "d38" distance of L2.end L40.end
  measures "d39" distance of L40.end L41.end
  measures "d40" distance of L40.end L43.end
  measures "d41" distance of L0.start L45.end
  measures "d42" distance of L45.end L46.end
  measures "d43" distance of L45.end L48.end
  measures "d44" distance of L34.end L50.end
  measures "d45" distance of L50.end L51.end
  measures "d46" distance of L50.end L53.end
  measures "d47" distance of L35.end L55.end
  measures "d48" distance of L55.end L56.end
  measures "d49" distance of L55.end L58.end
  measures "d50" distance of L36.end L60.end
  measures "d51" distance of L60.end L61.end
  measures "d52" distance of L60.end L63.end
  measures "d53" distance of L3 L37
extrude "Extrude3" add sketch "Sketch1" along normal blind 2 contours L0 L1 L2 L3 L4 L6 L7 L8 L9 L11 L12 L13 L14 L16 L17 L18 L19 L21 L22 L23 L24 L28 L29 L33 L34 L36 L37 L40 L41 L42 L43 L45 L46 L47 L48 L50 L52 L53 L54 L55 L57 L58 L59 L60 L61 L62 L63 | L1 L30 L31 L32 L33 | L1 L25 L26 L27 L28

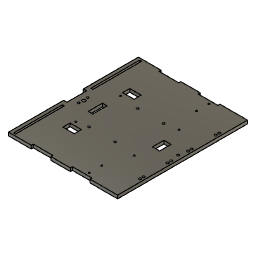
design "cage_front_200x168_trans_5mm"
Autodesk Fusion 360 part; units mm, degrees
sketch "Sketch1" plane through (0, 0, 0) normal (0, 0, 1) x (1, 0, 0)
  line L0 (0, 0) -> (168, 0)
  line L1 (168, 0) -> (168, -200)
  line L2 (168, -200) -> (0, -200)
  line L3 (0, -200) -> (0, 0)
  circle A0 centre (16, -100) radius 2.5
  line L4 (0, -200) -> (5, -200)
  line L5 (0, -197) -> (0, -200)
  line L6 (5, -197) -> (8, -197)
  line L7 (8, -197) -> (8, -122)
  line L8 (8, -122) -> (5, -122)
  line L9 (5, -122) -> (5, -197)
  line L10 (0, 0) -> (5, 0)
  line L11 (0, -3) -> (0, 0)
  line L12 (5, -3) -> (8, -3)
  line L13 (8, -3) -> (8, -78)
  line L14 (8, -78) -> (5, -78)
  line L15 (5, -78) -> (5, -3)
  circle A1 centre (15, -107) radius 1.6
  circle A2 centre (15, -93) radius 1.6
  circle A3 centre (128, -134.5) radius 1.25
  circle A4 centre (128, -65.5) radius 1.25
  circle A5 centre (38, -134.5) radius 1.25
  circle A6 centre (38, -65.5) radius 1.25
  circle A7 centre (108, -69) radius 1.6
  circle A8 centre (68, -69) radius 1.6
  circle A9 centre (55, -131) radius 1.6
  line L16 (33.75, -89) -> (40.75, -89)
  line L17 (40.75, -89) -> (40.75, -111)
  line L18 (40.75, -111) -> (33.75, -111)
  line L19 (33.75, -111) -> (33.75, -89)
  line L20 (33.75, -89) -> (40.75, -111) construction
  line L21 (40.75, -89) -> (33.75, -111) construction
  line L22 (84, -200) -> (116.5, -200)
  circle A10 centre (116.5, -192) radius 1.25
  circle A11 centre (116.5, -173) radius 1.25
  circle A12 centre (116.5, -8) radius 1.25
  circle A13 centre (116.5, -27) radius 1.25
  circle A14 centre (163.5, -39) radius 1.75
  circle A15 centre (163.5, -44.5) radius 1.75
  circle A16 centre (163.5, -81.5) radius 1.75
  circle A17 centre (163.5, -87) radius 1.75
  circle A18 centre (163.5, -39) radius 1.75
  circle A19 centre (163.5, -44.5) radius 1.75
  circle A20 centre (163.5, -81.5) radius 1.75
  circle A21 centre (163.5, -87) radius 1.75
  line L23 (168, -100) -> (161.6526, -100)
  circle A22 centre (163.5, -161) radius 1.75
  circle A23 centre (163.5, -155.5) radius 1.75
  circle A24 centre (163.5, -118.5) radius 1.75
  circle A25 centre (163.5, -113) radius 1.75
  line L24 (35.25, -59.5) -> (52.75, -59.5)
  line L25 (52.75, -59.5) -> (52.75, -48.5)
  line L26 (52.75, -48.5) -> (35.25, -48.5)
  line L27 (35.25, -48.5) -> (35.25, -59.5)
  line L28 (35.25, -59.5) -> (52.75, -48.5) construction
  line L29 (52.75, -59.5) -> (35.25, -48.5) construction
  line L30 (35.25, -151.5) -> (52.75, -151.5)
  line L31 (52.75, -151.5) -> (52.75, -140.5)
  line L32 (52.75, -140.5) -> (35.25, -140.5)
  line L33 (35.25, -140.5) -> (35.25, -151.5)
  line L34 (35.25, -151.5) -> (52.75, -140.5) construction
  line L35 (52.75, -151.5) -> (35.25, -140.5) construction
  line L36 (130.5, -108.75) -> (141.5, -108.75)
  line L37 (141.5, -108.75) -> (141.5, -91.25)
  line L38 (141.5, -91.25) -> (130.5, -91.25)
  line L39 (130.5, -91.25) -> (130.5, -108.75)
  line L40 (130.5, -108.75) -> (141.5, -91.25) construction
  line L41 (141.5, -108.75) -> (130.5, -91.25) construction
  circle A26 centre (95, -131) radius 1.6
  line L42 (-5.1, -115.1) -> (5.1, -115.1)
  line L43 (5.1, -115.1) -> (5.1, -84.9)
  line L44 (5.1, -84.9) -> (-5.1, -84.9)
  line L45 (-5.1, -84.9) -> (-5.1, -115.1)
  line L46 (-5.1, -115.1) -> (5.1, -84.9) construction
  line L47 (5.1, -115.1) -> (-5.1, -84.9) construction
  line L48 (0, 0) -> (35, 0)
  line L49 (35, 0) -> (65.2, 0)
  line L50 (65.2, 0) -> (65.2, -3.1)
  line L51 (65.2, -3.1) -> (35, -3.1)
  line L52 (35, -3.1) -> (35, 0)
  line L53 (65.2, 0) -> (95.2, 0)
  line L54 (95.2, 0) -> (125.4, 0)
  line L55 (125.4, 0) -> (125.4, -3.1)
  line L56 (125.4, -3.1) -> (95.2, -3.1)
  line L57 (95.2, -3.1) -> (95.2, 0)
  line L58 (0, -200) -> (35, -200)
  line L59 (35, -200) -> (65.2, -200)
  line L60 (65.2, -200) -> (65.2, -196.9)
  line L61 (65.2, -196.9) -> (35, -196.9)
  line L62 (35, -196.9) -> (35, -200)
  line L63 (65.2, -200) -> (95.2, -200)
  line L64 (95.2, -200) -> (125.4, -200)
  line L65 (125.4, -200) -> (125.4, -196.9)
  line L66 (125.4, -196.9) -> (95.2, -196.9)
  line L67 (95.2, -196.9) -> (95.2, -200)
  circle A27 centre (161.25, -100) radius 1.7
  point P0 (37.25, -100)
  point P1 (44, -54)
  point P2 (44, -146)
  point P3 (136, -100)
  point P4 (0, -100)
  dimension "d1" = 168
  dimension "d2" = 200
  dimension "d8" = 5
  dimension "d11" = 5
  dimension "d12" = 3
  dimension "d13" = 3
  dimension "d14" = 75
  dimension "d15" = 5
  dimension "d16" = 3
  dimension "d17" = 3
  dimension "d18" = 75
  dimension "d23" = 3.2
  dimension "d24" = 3.2
  dimension "d27" = 16
  dimension "d28" = 2.5
  dimension "d29" = 40
  dimension "d30" = 65.5
  dimension "d33" = 2.5
  dimension "d34" = 2.5
  dimension "d36" = 65.5
  dimension "d37" = 90
  dimension "d38" = 2.5
  dimension "d39" = 90
  dimension "d42" = 3.2
  dimension "d43" = 60
  dimension "d44" = 69
  dimension "d45" = 3.2
  dimension "d46" = 40
  dimension "d47" = 3.2
  dimension "d48" = 69
  dimension "d49" = 113
  dimension "d50" = 7
  dimension "d51" = 22
  dimension "d52" = 37.25
  dimension "d63" = 32.5
  dimension "d64" = 2.5
  dimension "d65" = 8
  dimension "d66" = 2.5
  dimension "d67" = 19
  dimension "d68" = 2.5
  dimension "d69" = 8
  dimension "d70" = 2.5
  dimension "d71" = 19
  dimension "d72" = 3.5
  dimension "d73" = 39
  dimension "d74" = 4.5
  dimension "d75" = 3.5
  dimension "d76" = 5.5
  dimension "d77" = 3.5
  dimension "d79" = 37
  dimension "d80" = 3.5
  dimension "d81" = 5.5
  dimension "d82" = 3.5
  dimension "d83" = 3.5
  dimension "d84" = 5.5
  dimension "d85" = 3.5
  dimension "d86" = 37
  dimension "d87" = 3.5
  dimension "d88" = 5.5
  dimension "d89" = 17.5
  dimension "d90" = 11
  dimension "d91" = 54
  dimension "d92" = 44
  dimension "d93" = 17.5
  dimension "d94" = 11
  dimension "d95" = 54
  dimension "d96" = 11
  dimension "d97" = 17.5
  dimension "d98" = 32
  dimension "d99" = 3.2
  dimension "d100" = 40
  dimension "d101" = 10.2
  dimension "d102" = 30.2
  dimension "d103" = 35
  dimension "d104" = 30.2
  dimension "d105" = 3.1
  dimension "d106" = 30
  dimension "d107" = 30.2
  dimension "d108" = 3.1
  dimension "d109" = 35
  dimension "d110" = 30.2
  dimension "d111" = 3.1
  dimension "d112" = 30
  dimension "d113" = 30.2
  dimension "d114" = 3.1
  dimension "d115" = 3.4
  dimension "d116" = 6.75
  constraint horizontal L0
  constraint vertical L1
  constraint horizontal L2
  constraint vertical L3
  constraint coincident L0.start L3.end
  constraint horizontal L4
  constraint vertical L5
  constraint horizontal L6
  constraint vertical L7
  constraint horizontal L8
  constraint vertical L9
  constraint horizontal L10
  constraint vertical L11
  constraint horizontal L12
  constraint vertical L13
  constraint horizontal L14
  constraint vertical L15
  constraint horizontal L16
  constraint perpendicular L16 L17
  constraint parallel L16 L18
  constraint parallel L17 L19
  constraint coincident L20 P0
  constraint coincident L21 P0
  constraint midpoint L2 L22.start
  constraint parallel L2 L22
  constraint midpoint L1 L23.start
  constraint perpendicular L1 L23
  constraint symmetric A14 L23 A22
  constraint symmetric A16 L23 A24
  constraint symmetric A17 L23 A25
  constraint symmetric A19 L23 A23
  constraint horizontal L24
  constraint perpendicular L24 L25
  constraint parallel L24 L26
  constraint parallel L25 L27
  constraint coincident L28 P1
  constraint coincident L29 P1
  constraint horizontal L30
  constraint perpendicular L30 L31
  constraint parallel L30 L32
  constraint parallel L31 L33
  constraint coincident L34 P2
  constraint coincident L35 P2
  constraint horizontal L36
  constraint perpendicular L36 L37
  constraint parallel L36 L38
  constraint parallel L37 L39
  constraint coincident L40 P3
  constraint coincident L41 P3
  constraint horizontal L42
  constraint perpendicular L42 L43
  constraint parallel L42 L44
  constraint parallel L43 L45
  constraint coincident L46 P4
  constraint coincident L47 P4
  constraint midpoint L3 P4
  constraint perpendicular L11 L48
  constraint horizontal L49
  constraint vertical L50
  constraint horizontal L51
  constraint vertical L52
  constraint perpendicular L50 L53
  constraint horizontal L54
  constraint vertical L55
  constraint horizontal L56
  constraint vertical L57
  constraint perpendicular L5 L58
  constraint horizontal L59
  constraint vertical L60
  constraint horizontal L61
  constraint vertical L62
  constraint perpendicular L60 L63
  constraint horizontal L64
  constraint vertical L65
  constraint horizontal L66
  constraint vertical L67
  measures "d1" distance of L0.start L0.end
  measures "d2" distance of L0.start L2.end
  measures "d8" diameter of A0
  measures "d11" distance of L2.end L4.end
  measures "d12" distance of L2.end L5.start
  measures "d13" distance of L6.start L6.end
  measures "d14" distance of L6.start L8.end
  measures "d15" distance of L0.start L10.end
  measures "d16" distance of L0.start L11.start
  measures "d17" distance of L12.start L12.end
  measures "d18" distance of L12.start L14.end
  measures "d23" diameter of A1
  measures "d24" diameter of A2
  measures "d27" distance of L3 A0.centre
  measures "d28" diameter of A3
  measures "d29" distance of L1 A3.centre
  measures "d30" distance of L2 A3.centre
  measures "d33" diameter of A4
  measures "d34" diameter of A5
  measures "d36" distance of L0 A4.centre
  measures "d37" distance of A3.centre A5.centre
  measures "d38" diameter of A6
  measures "d39" distance of A4.centre A6.centre
  measures "d42" diameter of A7
  measures "d43" distance of L1 A7.centre
  measures "d44" distance of L0 A7.centre
  measures "d45" diameter of A8
  measures "d46" distance of A7.centre A8.centre
  measures "d47" diameter of A9
  measures "d48" distance of L2 A9.centre
  measures "d49" distance of L1 A9.centre
  measures "d50" distance of L17.end L18.end
  measures "d51" distance of L16.end L17.end
  measures "d52" distance of L3 P0
  measures "d63" distance of L22.start L22.end
  measures "d64" diameter of A10
  measures "d65" distance of L22.end A10.centre
  measures "d66" diameter of A11
  measures "d67" distance of A10.centre A11.centre
  measures "d68" diameter of A12
  measures "d69" distance of L0 A12.centre
  measures "d70" diameter of A13
  measures "d71" distance of A12.centre A13.centre
  measures "d72" diameter of A14
  measures "d73" distance of L0 A14.centre
  measures "d74" distance of L1 A14.centre
  measures "d75" diameter of A15
  measures "d76" distance of A14.centre A15.centre
  measures "d77" diameter of A16
  measures "d79" distance of A15.centre A16.centre
  measures "d80" diameter of A17
  measures "d81" distance of A16.centre A17.centre
  measures "d82" diameter of A18
  measures "d83" diameter of A19
  measures "d84" distance of A14.centre A15.centre
  measures "d85" diameter of A20
  measures "d86" distance of A16.centre A15.centre
  measures "d87" diameter of A21
  measures "d88" distance of A16.centre A17.centre
  measures "d89" distance of L25.end L26.end
  measures "d90" distance of L24.end L25.end
  measures "d91" distance of L0 P1
  measures "d92" distance of L3 P1
  measures "d93" distance of L31.end L32.end
  measures "d94" distance of L30.end L31.end
  measures "d95" distance of L2 P2
  measures "d96" distance of L37.end L38.end
  measures "d97" distance of L36.end L37.end
  measures "d98" distance of L1 P3
  measures "d99" diameter of A26
  measures "d100" distance of A9.centre A26.centre
  measures "d101" distance of L43.end L44.end
  measures "d102" distance of L42.end L43.end
  measures "d103" distance of L0.start L48.end
  measures "d104" distance of L48.end L49.end
  measures "d105" distance of L48.end L51.end
  measures "d106" distance of L49.end L53.end
  measures "d107" distance of L53.end L54.end
  measures "d108" distance of L53.end L56.end
  measures "d109" distance of L2.end L58.end
  measures "d110" distance of L58.end L59.end
  measures "d111" distance of L58.end L61.end
  measures "d112" distance of L59.end L63.end
  measures "d113" distance of L63.end L64.end
  measures "d114" distance of L63.end L66.end
  measures "d115" diameter of A27
  measures "d116" distance of L1 A27.centre
extrude "Extrude7" add sketch "Sketch1" along normal blind 5 contours L0 L1 L2 L3 L4 L5 L10 L11 L22 L42 L43 L44 L48 L50 L51 L52 L53 L55 L56 L57 L58 L60 L61 L62 L63 L65 L66 L67
equation "d30 = ( 115 / 2 ) * 1 mm + 8 mm"
equation "d44 = ( 115 / 2 ) * 1 mm + 11.5 mm"

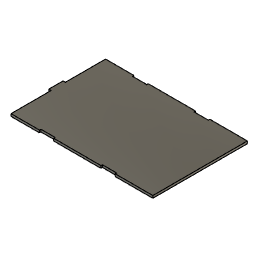
design "cage_bottom_305x200_blk_5mm"
Autodesk Fusion 360 part; units mm, degrees
sketch "Sketch1" plane through (0, 0, 0) normal (0, 0, 1) x (1, 0, 0)
  line L0 (0, 0) -> (300, 0)
  line L1 (300, 0) -> (300, -200)
  line L2 (300, -200) -> (0, -200)
  line L3 (0, -200) -> (0, 0)
  line L4 (0, 0) -> (60, 0)
  line L5 (60, 0) -> (90.2, 0)
  line L6 (90.2, 0) -> (90.2, -3.1)
  line L7 (90.2, -3.1) -> (60, -3.1)
  line L8 (60, -3.1) -> (60, 0)
  line L9 (90.2, 0) -> (190.2, 0)
  line L10 (190.2, 0) -> (220.4, 0)
  line L11 (220.4, 0) -> (220.4, -3.1)
  line L12 (220.4, -3.1) -> (190.2, -3.1)
  line L13 (190.2, -3.1) -> (190.2, 0)
  line L14 (0, -200) -> (60, -200)
  line L15 (60, -200) -> (90.2, -200)
  line L16 (90.2, -200) -> (90.2, -196.9)
  line L17 (90.2, -196.9) -> (60, -196.9)
  line L18 (60, -196.9) -> (60, -200)
  line L19 (90.2, -200) -> (190.2, -200)
  line L20 (190.2, -200) -> (220.4, -200)
  line L21 (220.4, -200) -> (220.4, -196.9)
  line L22 (220.4, -196.9) -> (190.2, -196.9)
  line L23 (190.2, -196.9) -> (190.2, -200)
  line L24 (0, 0) -> (0, -85)
  line L25 (0, -85) -> (-5, -85)
  line L26 (-5, -85) -> (-5, -115)
  line L27 (-5, -115) -> (0, -115)
  line L28 (0, -115) -> (0, -85)
  dimension "d1" = 300
  dimension "d2" = 200
  dimension "d5" = 60
  dimension "d6" = 30.2
  dimension "d7" = 3.1
  dimension "d8" = 100
  dimension "d9" = 30.2
  dimension "d10" = 3.1
  dimension "d11" = 60
  dimension "d12" = 30.2
  dimension "d13" = 3.1
  dimension "d14" = 100
  dimension "d15" = 30.2
  dimension "d16" = 3.1
  dimension "d17" = 85
  dimension "d18" = 30
  constraint horizontal L0
  constraint vertical L1
  constraint horizontal L2
  constraint vertical L3
  constraint coincident L0.start L3.end
  constraint perpendicular L3 L4
  constraint horizontal L5
  constraint vertical L6
  constraint horizontal L7
  constraint vertical L8
  constraint perpendicular L6 L9
  constraint horizontal L10
  constraint vertical L11
  constraint horizontal L12
  constraint vertical L13
  constraint perpendicular L3 L14
  constraint horizontal L15
  constraint vertical L16
  constraint horizontal L17
  constraint vertical L18
  constraint perpendicular L16 L19
  constraint horizontal L20
  constraint vertical L21
  constraint horizontal L22
  constraint vertical L23
  constraint coincident L3 L24.end
  constraint horizontal L25
  constraint vertical L26
  constraint horizontal L27
  constraint vertical L28
  measures "d1" distance of L0.start L0.end
  measures "d2" distance of L0.start L2.end
  measures "d5" distance of L0.start L4.end
  measures "d6" distance of L4.end L5.end
  measures "d7" distance of L4.end L7.end
  measures "d8" distance of L5.end L9.end
  measures "d9" distance of L9.end L10.end
  measures "d10" distance of L9.end L12.end
  measures "d11" distance of L2.end L14.end
  measures "d12" distance of L14.end L15.end
  measures "d13" distance of L14.end L17.end
  measures "d14" distance of L15.end L19.end
  measures "d15" distance of L19.end L20.end
  measures "d16" distance of L19.end L22.end
  measures "d17" distance of L0.start L24.end
  measures "d18" distance of L24.end L27.end
extrude "Extrude1" add sketch "Sketch1" along normal blind 5 contours L0 L1 L2 L3 L4 L6 L7 L8 L9 L11 L12 L13 L14 L16 L17 L18 L19 L21 L22 L23 L24 L28 | L3 L25 L26 L27 L28

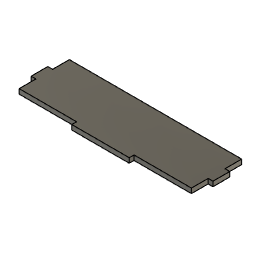
design "tray_front_76x23_trans_2mm"
Autodesk Fusion 360 part; units mm, degrees